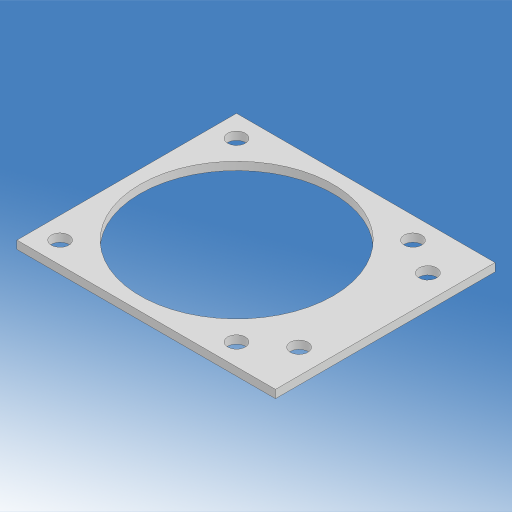
# Autodesk Inventor part: MotorPlate
Saved by Autodesk Inventor 2024 (Build 280153000, 153)
## iProperties
Created: 2024-02-28
Part Number: MotorPlate
Material: Generic
Document SubType Name: Modeling
Designer: seene
Density: 1 g/cm^3
Appearance: Default
Author: seene
Autodesk Inventor part; units mm, degrees
ref_plane "YZ Plane" through (0, 0, 0) normal (1, 0, 0) x (0, 1, 0)
ref_plane "XZ Plane" through (0, 0, 0) normal (0, 1, 0) x (-1, 0, 0)
ref_plane "XY Plane" through (0, 0, 0) normal (0, 0, 1) x (1, 0, 0)
sketch "Sketch1" plane through (0, 0, 0) normal (0, 1, 0) x (-1, 0, 0)
  line L0 (0, 0) -> (-101.981, 0)
  line L1 (-101.981, 0) -> (-101.981, -86.614)
  line L2 (-101.981, -86.614) -> (0, -86.614)
  line L3 (0, -86.614) -> (0, 0)
  circle A0 centre (-8.5085, -8.5085) radius 3.4925
  circle A1 centre (-78.1055, -8.5085) radius 3.4925
  circle A2 centre (-8.5085, -78.1055) radius 3.4925
  circle A3 centre (-78.1055, -78.1055) radius 3.4925
  circle A4 centre (-43.3338, -43.3338) radius 38.1
  circle A5 centre (-92.2419, -19.05) radius 3.5
  circle A6 centre (-92.2419, -69.85) radius 3.5
  dimension "d0" = 101.981
  dimension "d1" = 86.614
  dimension "d2" = 6.985
  dimension "d3" = 8.5085
  dimension "d4" = 8.5085
  dimension "d7" = 69.597
  dimension "d10" = 69.597
  dimension "d13" = 76.2
  dimension "d14" = 43.3338
  dimension "d15" = 43.3338
  dimension "d16" = 7
  dimension "d19" = 50.8
  dimension "d24" = 19.05
  constraints: 8 end point, 7 centre point, 2 horizontal, 2 parallel, 2 vertical, 1 perpendicular, 8 other
  measures "d0" distance of L1.end L2.end
  measures "d1" distance of L0.end L1.end
  measures "d2" diameter of A0
  measures "d3" distance from line of L3 A0.centre
  measures "d4" distance from line of L0 A0.centre
  measures "d7" distance of A0.centre A1.centre
  measures "d10" distance of A0.centre A2.centre
  measures "d13" diameter of A4
  measures "d14" distance from line of L3 A4.centre
  measures "d15" distance from line of L0 A4.centre
  measures "d16" diameter of A5
  measures "d19" distance of A5.centre A6.centre
  measures "d24" distance from line of A5.centre L0
extrude "Extrusion1" add sketch "Sketch1" along normal blind 3.175
body "Solid1"
